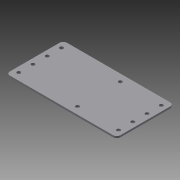
# Autodesk Inventor part: Motor Mount
Saved by Autodesk Inventor 2014 (Build 180170000, 170)
## iProperties
Created: 2015-01-20
Part Number: Motor Mount
Material: Generic
Document SubType Name: Sheet Metal
Designer: chappelled
Density: 1 g/cm^3
Sheet Metal Rule: Default
Appearance: Default
Author: chappelled
Autodesk Inventor part; units mm, degrees
ref_plane "YZ Plane" through (0, 0, 0) normal (1, 0, 0) x (0, 1, 0)
ref_plane "XZ Plane" through (0, 0, 0) normal (0, 1, 0) x (-1, 0, 0)
ref_plane "XY Plane" through (0, 0, 0) normal (0, 0, 1) x (1, 0, 0)
sketch "Sketch1" plane through (0, 0, 0) normal (0, 1, 0) x (-1, 0, 0)
  line L0 (0, 0) -> (-196.85, 0)
  line L1 (-196.85, 0) -> (-196.85, 101.6)
  line L2 (-196.85, 101.6) -> (0, 101.6)
  line L3 (0, 101.6) -> (0, 0)
  dimension "d0" = 196.85
  dimension "d1" = 101.6
  measures "d0" distance of L1.end L2.end
  measures "d1" distance of L0.end L1.end
extrude "Plate1" add sketch "Sketch1" along normal blind 3.175
hole "Hole1" at (9.525, 3.175, 12.7) direction (0, -1, 0) diameter 6.35 end through all
hole "Hole2" at (187.325, 3.175, 12.7) direction (0, -1, 0) diameter 6.35 end through all
pattern_linear "Rectangular Pattern1" count 4 spacing 25.4 along (0, 0, 1) of "Hole1"
pattern_linear "Rectangular Pattern2" count 4 spacing 25.4 along (0, 0, 1) of "Hole2"
fillet "Fillet1" radius 6.35 1 edges at (0, 1.5875, 101.6)
fillet "Fillet2" radius 6.35 1 edges at (0, 1.5875, 0)
fillet "Fillet3" radius 6.35 1 edges at (196.85, 1.5875, 101.6)
fillet "Fillet4" radius 6.35 1 edges at (196.85, 1.5875, 0)
hole "Hole3" at (114.3, 3.175, 12.7) direction (0, -1, 0) diameter 6.35 end through all
pattern_linear "Rectangular Pattern3" count 2 spacing 76.2 along (0, 0, 1) of "Hole3"
equation "\"d10\" = Thickness"
equation "\"d19\" = Thickness"
equation "\"d38\" = Thickness"
equation "\"BendRadius\" = Thickness"
equation "\"BendReliefWidth\" = Thickness"
equation "\"BendReliefDepth\" = 0.5 * Thickness"
equation "\"CornerReliefSize\" = 4 * Thickness"
equation "\"MinimumRemnant\" = 2 * Thickness"
equation "\"TransitionRadius\" = BendRadius"
equation "\"JacobiRadiusSize\" = BendRadius"
equation "\"GapSize\" = Thickness"
equation "\"d2\" = BendRadius"
equation "\"Thickness\" = 3.175"
body "Solid1"
